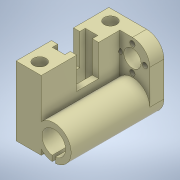
# Autodesk Inventor part: xaxissupport1
Saved by Autodesk Inventor 2020.2 (Build 242310000, 310)
## iProperties
Created: 2017-10-26
Part Number: xaxissupport1
Material: Polipropylen
Document SubType Name: Modeling
Designer: wojte
Density: 0.899 g/cm^3
Appearance: Gładki - popielaty
Author: wojte
Autodesk Inventor part; units mm, degrees
ref_plane "YZ Plane" through (0, 0, 0) normal (1, 0, 0) x (0, 1, 0)
ref_plane "XZ Plane" through (0, 0, 0) normal (0, 1, 0) x (-1, 0, 0)
ref_plane "XY Plane" through (0, 0, 0) normal (0, 0, 1) x (1, 0, 0)
sketch "Szkic1" plane through (0, 0, 0) normal (0, 1, 0) x (-1, 0, 0)
  line L0 (0, 0) -> (16, 0)
  line L1 (16, 0) -> (16, -44)
  line L2 (16, -44) -> (0, -44)
  line L3 (0, -44) -> (0, 0)
  dimension "d0" = 44
  dimension "d1" = 16
  constraints: 8 end point, 2 parallel, 1 horizontal, 1 perpendicular
  measures "d0" distance of L0.end L1.end
  measures "d1" distance of L0.start L0.end
extrude "Wyciągnięcie proste1" add sketch "Szkic1" along normal blind 59
sketch "Szkic2" plane through (0, 59, 0) normal (0, 1, 0) x (1, 0, 0)
  line L0 (0, 44) -> (19, 44)
  line L1 (19, 44) -> (19, 0)
  line L2 (19, 0) -> (0, 0)
  line L3 (0, 0) -> (0, 44)
  dimension "d4" = 19
  constraints: 8 end point, 2 parallel, 2 point on line, 1 coincident, 1 horizontal, 1 perpendicular
  measures "d4" distance of L0.start L0.end
extrude "Wyciągnięcie proste2" add sketch "Szkic2" against normal blind 9
fillet "Zaokrąglenie1" radius 11 2 edges at (19, 54.5, 0) (19, 54.5, -44)
sketch "Szkic3" plane through (0, 59, 0) normal (0, 1, 0) x (1, 0, 0)
  arc A0 (8, 0) -> (19, 11) centre (8, 11) ccw projected
  point P0 (0, 0)
  constraints: 1 coincident
hole "Otwór1" at (8, 59, -11) direction (0, -1, 0) diameter 15 end through all
sketch "Szkic4" plane through (0, 59, 0) normal (0, 1, 0) x (1, 0, 0)
  arc A0 (19, 33) -> (8, 44) centre (8, 33) ccw projected
  point P0 (0, 0)
  point P1 (8, 32.5)
  dimension "d85" = 0.5
  constraints: 1 vertical alignment
  measures "d85" distance of A0.centre point (8, 32.5)
hole "Otwór2" at (8, 59, -32.5) direction (0, -1, 0) diameter 11 end through all
sketch "Szkic5" plane through (0, 59, 0) normal (0, 1, 0) x (1, 0, 0)
  circle A0 centre (8, 32.5) radius 5.5 projected
  point P0 (0, 0)
  point P1 (8, 24.5)
  point P2 (16, 32.5)
  point P3 (8, 40.5)
  point P4 (0, 32.5)
  dimension "d23" = 8
  dimension "d26" = 360
  constraints: 1 vertical alignment, 5 other
  measures "d23" distance of A0.centre point (8, 24.5)
hole "Otwór3" at (8, 59, -24.5) at (16, 59, -32.5) at (8, 59, -40.5) at (0, 59, -32.5) direction (0, -1, 0) diameter 3.4 depth 9 tip angle 118
sketch "Szkic6" plane through (0, 50, 0) normal (0, -1, 0) x (1, 0, 0)
  arc A0 (19, -11) -> (8, 0) centre (8, -11) ccw projected
  arc A1 (7, -0.0455) -> (9, -0.0455) centre (8, -11) ccw
  line L0 (8, -11) -> (8, 0) construction
  line L1 (9, -3.567) -> (9, 0)
  line L2 (7, -3.567) -> (7, 0)
  circle A2 centre (8, -11) radius 7.5 projected
  point P0 (0, 0)
  dimension "d35" = 22
  dimension "d36" = 2
  constraints: 6 end point, 4 point on circle, 2 parallel, 2 point on line, 1 centre point, 1 coincident, 1 vertical, 1 other
  measures "d35" diameter of A1
  measures "d36" distance between parallel lines of L2 L1
extrude "Wyciągnięcie proste3" add sketch "Szkic6" along normal up to surface (50 mm away) contours A1 L2 A2 L1 A0
sketch "Szkic11" plane through (0, 0, -44) normal (0, 0, -1) x (-1, 0, 0)
  line L0 (12, 19) -> (4, 19)
  line L1 (4, 19) -> (4, 40)
  line L2 (4, 40) -> (12, 40)
  line L3 (12, 40) -> (12, 19)
  line L4 (-8, 59) -> (16, 59) projected
  line L5 (0, 0) -> (16, 0) projected
  line L6 (8, 0) -> (8, 59) construction
  dimension "d68" = 8
  dimension "d69" = 21
  dimension "d70" = 19
  constraints: 10 end point, 2 parallel, 1 horizontal, 1 midpoint, 1 perpendicular, 1 point on line, 1 vertical, 1 other
  measures "d68" distance of L1.end L2.end
  measures "d69" distance of L0.end L1.end
  measures "d70" distance between parallel lines of L4 L2
extrude "Wyciągnięcie proste7" cut sketch "Szkic11" against normal through all
sketch "Szkic12" plane through (0, 0, -44) normal (0, 0, -1) x (-1, 0, 0)
  line L0 (4, 19) -> (4, 40) projected
  line L1 (12, 40) -> (12, 19) projected
  line L2 (0, 0) -> (0, 50) projected
  line L3 (-8, 59) -> (16, 59) projected
  line L4 (4, 40) -> (12, 40) projected
  line L5 (12, 19) -> (4, 19) projected
  point P0 (8, 52)
  point P1 (8, 7)
  dimension "d73" = 8
  dimension "d76" = 12
  dimension "d77" = 12
  constraints: 1 vertical alignment
  measures "d73" distance from line of point (8, 52) L2
  measures "d76" distance from line of L4 point (8, 52)
  measures "d77" distance from line of L5 point (8, 7)
hole "Otwór6" at (-8, 52, -44) at (-8, 7, -44) direction (0, 0, 1) diameter 8 end through all
ref_plane "Płaszczyzna konstrukcyjna1" through (0, 0, -54) normal (0, 0, -1) x (-1, 0, 0)
mirror "Odbij1" about plane through (0, 0, -54) normal (0, 0, -1) remove original yes
sketch "Szkic13" plane through (-16, 0, -108) normal (-1, 0, 0) x (0, 0, 1)
  line L0 (24, 36.5) -> (44, 36.5)
  line L1 (44, 36.5) -> (44, 22.5)
  line L2 (44, 22.5) -> (24, 22.5)
  line L3 (24, 22.5) -> (24, 36.5)
  line L4 (44, 0) -> (44, 59) projected
  point P0 (108, 0)
  point P1 (24, 29.5)
  point P2 (44, 29.5)
  dimension "d89" = 14
  dimension "d90" = 20
  constraints: 8 end point, 3 midpoint, 1 horizontal, 1 parallel, 1 perpendicular, 1 vertical
  measures "d89" distance of L0.end L1.end
  measures "d90" distance of L1.end L2.end
extrude "Wyciągnięcie proste8" cut sketch "Szkic13" against normal through all
thread "Gwint1" size "M3.5x0.6" class "6H" standard "ANSI Metric M Profile" full length
thread "Gwint2" size "M3.5x0.6" class "6H" standard "ANSI Metric M Profile" full length
thread "Gwint3" size "M3.5x0.6" class "6H" standard "ANSI Metric M Profile" full length
thread "Gwint4" size "M3.5x0.6" class "6H" standard "ANSI Metric M Profile" full length
